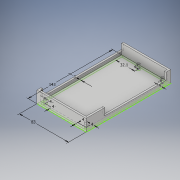
# Autodesk Inventor part: rumba_frame_mount
Saved by Autodesk Inventor 2019.1 (Build 231200000, 200)
## iProperties
Created: 2018-07-25
Part Number: rumba_frame_mount
Material: Generic
Document SubType Name: Modeling
Designer: verdammte
Density: 1 g/cm^3
Appearance: Default
Author: verdammte
Autodesk Inventor part; units mm, degrees
ref_plane "YZ Plane" through (0, 0, 0) normal (1, 0, 0) x (0, 1, 0)
ref_plane "XZ Plane" through (0, 0, 0) normal (0, 1, 0) x (-1, 0, 0)
ref_plane "XY Plane" through (0, 0, 0) normal (0, 0, 1) x (1, 0, 0)
sketch "Sketch1" plane through (0, 0, 0) normal (0, 1, 0) x (-1, 0, 0)
  line L0 (32.5791, 64.9096) -> (-50.4209, 64.9096)
  line L1 (-50.4209, 64.9096) -> (-50.4209, -78.0904)
  line L2 (-50.4209, -78.0904) -> (32.5791, -78.0904)
  line L3 (32.5791, -78.0904) -> (32.5791, 64.9096)
  line L4 (29.5791, 61.9096) -> (-47.4209, 61.9096)
  line L5 (-47.4209, 61.9096) -> (-47.4209, -75.0904)
  line L6 (-47.4209, -75.0904) -> (29.5791, -75.0904)
  line L7 (29.5791, -75.0904) -> (29.5791, 61.9096)
  line L8 (29.5791, -75.0904) -> (29.5791, -78.0904)
  line L9 (-47.4209, -70.2006) -> (-50.4209, -70.2006)
  line L10 (-47.4209, 33.4969) -> (-50.4209, 33.4969)
  line L11 (29.5791, 57.9608) -> (32.5791, 57.9608)
  point P0 (0, 0)
  dimension "d0" = 143
  dimension "d1" = 83
  dimension "d2" = 3
  constraints: 24 end point, 8 point on line, 5 perpendicular, 4 parallel, 1 horizontal, 3 other
  measures "d0" distance of L2.end L0.start
  measures "d1" distance of L0.start L0.end
  measures "d2" distance between parallel lines of L3 L7
extrude "Floor" add sketch "Sketch1" along normal blind 3
extrude "Walls" add sketch "Sketch1" along normal blind 20 contours L3 L11 L7 L4 L5 L10 L1 L0 | L3 L2 L8 L7 L11 | L10 L5 L9 L1 | L9 L5 L6 L8 L2 L1
sketch "Sketch2" plane through (0, 0, 0) normal (0, 1, 0) x (-1, 0, 0)
  line L0 (-47.4209, 61.9096) -> (29.5791, 61.9096) projected
  line L1 (29.5791, -75.0904) -> (-47.4209, -75.0904) projected
  line L2 (29.5791, 61.9096) -> (29.5791, -75.0904) projected
  line L3 (-47.4209, -75.0904) -> (-47.4209, 61.9096) projected
  circle A0 centre (25.5791, 57.9096) radius 2.5
  circle A1 centre (-43.4209, 57.9096) radius 2.5
  circle A2 centre (-43.4209, -71.0904) radius 2.5
  circle A3 centre (-2.5209, -71.0904) radius 2.5
  line L4 (-47.4209, 61.9096) -> (-47.4209, -75.0904) projected
  line L5 (-47.4209, -68.5904) -> (-50.4209, -68.5904)
  line L6 (-50.4209, -68.5904) -> (-50.4209, 27.9367)
  line L7 (-50.4209, 64.9096) -> (-50.4209, -78.0904) projected
  line L8 (-47.4209, 27.9367) -> (-50.4209, 27.9367)
  line L9 (29.5791, -75.0904) -> (29.5791, 61.9096) projected
  line L10 (29.5791, 55.4096) -> (32.4454, 55.4096)
  line L11 (-47.4209, -75.0904) -> (29.5791, -75.0904) projected
  line L12 (29.5791, -75.0904) -> (29.5791, -78.0904)
  point P0 (0, 0)
  dimension "d30" = 4
  dimension "d31" = 4
  dimension "d32" = 4
  dimension "d33" = 4
  dimension "d34" = 4
  dimension "d35" = 4
  dimension "d36" = 4
  dimension "d37" = 32.1
  constraints: 10 end point, 4 centre point, 4 coincident, 4 point on line, 2 horizontal, 1 perpendicular, 1 vertical
  measures "d30" distance from line of L0 A0.centre
  measures "d31" distance from line of L0 A1.centre
  measures "d32" distance from line of L1 A2.centre
  measures "d33" distance from line of L1 A3.centre
  measures "d34" distance from line of L2 A0.centre
  measures "d35" distance from line of L3 A1.centre
  measures "d36" distance from line of L3 A2.centre
  measures "d37" distance from line of L2 A3.centre
extrude "mounts" add sketch "Sketch2" along normal blind 8 contours A0 | A1 | A2 | A3
hole "Hole1" at (43.4209, 0, -71.0904) at (43.4209, 0, 57.9096) at (2.5209, 0, -71.0904) at (-25.5791, 0, 57.9096) direction (0, 1, 0) diameter 3 depth 8
extrude "Extrusion5" cut sketch "Sketch1" along normal blind 20 contours L10 L5 L9 L1
extrude "Extrusion6" cut sketch "Sketch1" along normal blind 20 contours L3 L2 L8 L7 L11
extrude "Extrusion7" add sketch "Sketch1" along normal blind 8 contours L10 L5 L9 L1
extrude "Extrusion8" add sketch "Sketch1" along normal blind 8 contours L3 L2 L8 L7 L11
body "Solid1"
